Autodesk Fusion 360 part; units mm, degrees
note: some values were not read from the file. Chosen so that the rebuilt part matches the saved one: which bodies a step acts on. Set by a fixed rule: which sketch regions a step uses.
(part 2 of 3)
  line L946 (0.5127, -14.5835) -> (0.5127, -14.573)
  line L947 (0.9043, -14.7211) -> (1.0101, -14.52)
  line L948 (0.5074, -14.5941) -> (0.4915, -14.6153)
  line L949 (0.4915, -14.6153) -> (0.4809, -14.6259)
  line L950 (0.4809, -14.6259) -> (0.4598, -14.6312)
  line L951 (0.4598, -14.6312) -> (0.4439, -14.6206)
  line L952 (0.4439, -14.6206) -> (0.4227, -14.6047)
  line L953 (0.8778, -14.6047) -> (0.899, -14.5888)
  line L954 (0.899, -14.5888) -> (0.9148, -14.5677)
  line L955 (0.8778, -14.6047) -> (0.8566, -14.6259)
  line L956 (0.8566, -14.6259) -> (0.8355, -14.6312)
  line L957 (0.8355, -14.6312) -> (0.8196, -14.6259)
  line L958 (0.8196, -14.6259) -> (0.809, -14.6153)
  line L959 (0.809, -14.6153) -> (0.7931, -14.5941)
  line L960 (0.9043, -14.7211) -> (0.7296, -14.7211)
  line L961 (0.5709, -14.7211) -> (0.3963, -14.7211)
  line L962 (1.0101, -14.52) -> (0.9783, -14.52)
  line L963 (0.7138, -14.52) -> (0.5868, -14.52)
  line L964 (0.3222, -14.52) -> (0.2904, -14.52)
  line L965 (0.9783, -14.52) -> (0.9677, -14.52)
  line L966 (0.9677, -14.52) -> (0.9519, -14.5306)
  line L967 (0.9519, -14.5306) -> (0.9148, -14.5677)
  line L968 (0.5868, -14.52) -> (0.5656, -14.52)
  line L969 (0.5656, -14.52) -> (0.5444, -14.5306)
  line L970 (0.5444, -14.5306) -> (0.5127, -14.573)
  line L971 (14.0223, -13.8004) -> (14.0223, -14.0755)
  line L972 (14.0223, -14.2396) -> (14.0223, -14.52)
  line L973 (13.9905, -14.52) -> (13.9905, -14.2396)
  line L974 (13.9905, -14.0755) -> (13.9905, -13.8004)
  line L975 (13.9323, -14.5677) -> (13.9323, -14.266)
  line L976 (13.9323, -14.102) -> (13.9323, -13.8004)
  line L977 (13.8953, -14.6047) -> (13.8953, -14.2872)
  line L978 (13.8953, -14.1232) -> (13.8953, -13.8004)
  line L979 (13.8106, -14.5941) -> (13.8106, -14.2766)
  line L980 (13.8106, -14.1179) -> (13.8106, -13.8004)
  line L981 (13.8, -13.8004) -> (13.8, -14.1073)
  line L982 (13.8, -14.266) -> (13.8, -14.573)
  line L983 (13.599, -14.52) -> (13.599, -14.2396)
  line L984 (13.599, -14.0755) -> (13.599, -13.8004)
  line L985 (13.9218, -14.7211) -> (14.0223, -14.52)
  line L986 (13.5302, -14.573) -> (13.5196, -14.5941)
  line L987 (13.5302, -14.573) -> (13.5302, -14.266)
  line L988 (13.5302, -14.1073) -> (13.5302, -13.8004)
  line L989 (13.5196, -14.5941) -> (13.5196, -14.2766)
  line L990 (13.5196, -14.1179) -> (13.5196, -13.8004)
  line L991 (13.4349, -14.6047) -> (13.4349, -14.2872)
  line L992 (13.4349, -14.1232) -> (13.4349, -13.8004)
  line L993 (13.3979, -13.8004) -> (13.3979, -14.102)
  line L994 (13.3979, -14.266) -> (13.3979, -14.5677)
  line L995 (13.3397, -13.8004) -> (13.3397, -14.0755)
  line L996 (13.3397, -14.2396) -> (13.3397, -14.52)
  line L997 (13.3079, -13.8004) -> (13.3079, -14.0755)
  line L998 (13.3079, -14.2396) -> (13.3079, -14.52)
  line L999 (13.9323, -14.5677) -> (13.9482, -14.5465)
  line L1000 (13.9482, -14.5465) -> (13.9641, -14.5306)
  line L1001 (13.9641, -14.5306) -> (13.98, -14.52)
  line L1002 (13.98, -14.52) -> (13.9905, -14.52)
  line L1003 (13.9323, -14.5677) -> (13.8953, -14.6047)
  line L1004 (13.5302, -14.573) -> (13.5407, -14.5518)
  line L1005 (13.5407, -14.5518) -> (13.5566, -14.5306)
  line L1006 (13.5566, -14.5306) -> (13.5778, -14.52)
  line L1007 (13.5778, -14.52) -> (13.599, -14.52)
  line L1008 (13.8106, -14.5941) -> (13.8, -14.573)
  line L1009 (13.4085, -14.7211) -> (13.3079, -14.52)
  line L1010 (13.8106, -14.5941) -> (13.8212, -14.6153)
  line L1011 (13.8212, -14.6153) -> (13.8371, -14.6259)
  line L1012 (13.8371, -14.6259) -> (13.853, -14.6312)
  line L1013 (13.853, -14.6312) -> (13.8741, -14.6206)
  line L1014 (13.8741, -14.6206) -> (13.8953, -14.6047)
  line L1015 (13.4349, -14.6047) -> (13.3979, -14.5677)
  line L1016 (13.4349, -14.6047) -> (13.4561, -14.6259)
  line L1017 (13.4561, -14.6259) -> (13.4773, -14.6312)
  line L1018 (13.4773, -14.6312) -> (13.4931, -14.6259)
  line L1019 (13.4931, -14.6259) -> (13.509, -14.6153)
  line L1020 (13.509, -14.6153) -> (13.5196, -14.5941)
  line L1021 (13.4085, -14.7211) -> (13.5831, -14.7211)
  line L1022 (13.7471, -14.7211) -> (13.9218, -14.7211)
  line L1023 (13.3079, -14.52) -> (13.3397, -14.52)
  line L1024 (13.599, -14.52) -> (13.7313, -14.52)
  line L1025 (13.9905, -14.52) -> (14.0223, -14.52)
  line L1026 (13.3397, -14.52) -> (13.3503, -14.52)
  line L1027 (13.3503, -14.52) -> (13.3979, -14.5677)
  line L1028 (13.7313, -14.52) -> (13.7524, -14.52)
  line L1029 (13.7524, -14.52) -> (13.7683, -14.5306)
  line L1030 (13.7683, -14.5306) -> (13.7895, -14.5518)
  line L1031 (13.7895, -14.5518) -> (13.8, -14.573)
  line L1032 (0.5285, -0.3807) -> (0.5285, -0.3966)
  line L1033 (0.5285, -0.3966) -> (0.5233, -0.4019)
  line L1034 (0.5233, -0.4019) -> (0.5233, -0.4178)
  line L1035 (0.5233, -0.4178) -> (0.518, -0.4178)
  line L1036 (0.518, -0.4178) -> (0.518, -0.4283)
  line L1037 (0.518, -0.4283) -> (0.5127, -0.4336)
  line L1038 (0.4809, -0.4707) -> (0.4756, -0.4707)
  line L1039 (0.4756, -0.4707) -> (0.4703, -0.476)
  line L1040 (0.4703, -0.476) -> (0.4598, -0.476)
  line L1041 (0.4598, -0.476) -> (0.4598, -0.4813)
  line L1042 (0.4598, -0.4813) -> (0.4386, -0.4813)
  line L1043 (0.4386, -0.4813) -> (0.4333, -0.4865)
  line L1044 (0.4333, -0.4865) -> (0.4227, -0.4865)
  line L1045 (0.5285, -0.3648) -> (0.5285, -0.3807)
  line L1046 (0.5285, -0.3648) -> (0.5285, -0.349)
  line L1047 (0.5285, -0.349) -> (0.5338, -0.3437)
  line L1048 (0.5338, -0.3437) -> (0.5338, -0.3384)
  line L1049 (0.5338, -0.3384) -> (0.5391, -0.3384)
  line L1050 (0.5391, -0.3384) -> (0.5391, -0.3331)
  line L1051 (0.5391, -0.3331) -> (0.5444, -0.3278)
  line L1052 (0.5444, -0.3278) -> (0.5497, -0.3225)
  line L1053 (0.5497, -0.3225) -> (0.555, -0.3225)
  line L1054 (0.555, -0.3225) -> (0.555, -0.3172)
  line L1055 (0.555, -0.3172) -> (0.5656, -0.3172)
  line L1056 (0.7349, -0.3172) -> (0.6767, -0.3066)
  line L1057 (0.6238, -0.3066) -> (0.5656, -0.3172)
  line L1058 (0.7349, -0.3172) -> (0.7455, -0.3172)
  line L1059 (0.7455, -0.3172) -> (0.7455, -0.3225)
  line L1060 (0.7455, -0.3225) -> (0.7561, -0.3225)
  line L1061 (0.7561, -0.3225) -> (0.7561, -0.3278)
  line L1062 (0.7561, -0.3278) -> (0.7614, -0.3331)
  line L1063 (0.7614, -0.3331) -> (0.7667, -0.3331)
  line L1064 (0.7667, -0.3331) -> (0.7667, -0.3437)
  line L1065 (0.7667, -0.3437) -> (0.772, -0.349)
  line L1066 (0.772, -0.349) -> (0.772, -0.3648)
  line L1067 (0.772, -0.3807) -> (0.772, -0.3648)
  line L1068 (0.8778, -0.4865) -> (0.8672, -0.4865)
  line L1069 (0.8672, -0.4865) -> (0.8619, -0.4812)
  line L1070 (0.8619, -0.4812) -> (0.8408, -0.4812)
  line L1071 (0.8408, -0.4812) -> (0.8408, -0.476)
  line L1072 (0.8408, -0.476) -> (0.8302, -0.476)
  line L1073 (0.8302, -0.476) -> (0.8302, -0.4707)
  line L1074 (0.8302, -0.4707) -> (0.8196, -0.4707)
  line L1075 (0.7878, -0.4336) -> (0.7878, -0.4283)
  line L1076 (0.7878, -0.4283) -> (0.7825, -0.4283)
  line L1077 (0.7825, -0.4283) -> (0.7825, -0.4177)
  line L1078 (0.7825, -0.4177) -> (0.7773, -0.4177)
  line L1079 (0.7773, -0.4177) -> (0.7773, -0.4019)
  line L1080 (0.7773, -0.4019) -> (0.772, -0.3966)
  line L1081 (0.772, -0.3966) -> (0.772, -0.3807)
  line L1082 (0.8937, -0.4865) -> (0.8778, -0.4865)
  line L1083 (0.8937, -0.4865) -> (0.9254, -0.4865)
  line L1084 (0.9254, -0.4865) -> (0.9254, -0.4918)
  line L1085 (0.9254, -0.4918) -> (0.936, -0.4918)
  line L1086 (0.936, -0.4918) -> (0.9413, -0.4971)
  line L1087 (0.9413, -0.4971) -> (0.9466, -0.4971)
  line L1088 (0.9466, -0.4971) -> (0.9519, -0.5024)
  line L1089 (0.9519, -0.5024) -> (0.9572, -0.5024)
  line L1090 (0.9572, -0.5024) -> (0.9572, -0.5077)
  line L1091 (0.9572, -0.5077) -> (0.9625, -0.5077)
  line L1092 (0.9625, -0.5077) -> (0.9625, -0.513)
  line L1093 (0.9625, -0.513) -> (0.9678, -0.513)
  line L1094 (0.9678, -0.513) -> (0.9678, -0.5183)
  line L1095 (0.9678, -0.5183) -> (0.973, -0.5183)
  line L1096 (0.973, -0.5183) -> (0.973, -0.5236)
  line L1097 (0.973, -0.5236) -> (0.9783, -0.5236)
  line L1098 (0.9783, -0.5236) -> (0.9783, -0.5289)
  line L1099 (0.9783, -0.5289) -> (0.9836, -0.5342)
  line L1100 (0.9836, -0.5342) -> (0.9836, -0.5395)
  line L1101 (0.9836, -0.5395) -> (0.9889, -0.5395)
  line L1102 (0.9889, -0.5395) -> (0.9889, -0.55)
  line L1103 (0.9889, -0.55) -> (0.9942, -0.5553)
  line L1104 (0.9942, -0.7723) -> (1.0048, -0.7194)
  line L1105 (1.0048, -0.7194) -> (1.0048, -0.6876)
  line L1106 (1.0048, -0.64) -> (1.0048, -0.6083)
  line L1107 (1.0048, -0.6083) -> (0.9942, -0.5553)
  line L1108 (0.9942, -0.7723) -> (0.9889, -0.7776)
  line L1109 (0.9889, -0.7776) -> (0.9889, -0.7882)
  line L1110 (0.9889, -0.7882) -> (0.9836, -0.7882)
  line L1111 (0.9836, -0.7882) -> (0.9836, -0.7935)
  line L1112 (0.9836, -0.7935) -> (0.9783, -0.7988)
  line L1113 (0.9783, -0.7988) -> (0.9783, -0.804)
  line L1114 (0.9783, -0.804) -> (0.973, -0.804)
  line L1115 (0.973, -0.804) -> (0.973, -0.8093)
  line L1116 (0.973, -0.8093) -> (0.9677, -0.8093)
  line L1117 (0.9677, -0.8093) -> (0.9677, -0.8146)
  line L1118 (0.9677, -0.8146) -> (0.9625, -0.8146)
  line L1119 (0.9625, -0.8146) -> (0.9625, -0.8199)
  line L1120 (0.9625, -0.8199) -> (0.9572, -0.8199)
  line L1121 (0.9572, -0.8199) -> (0.9572, -0.8252)
  line L1122 (0.9572, -0.8252) -> (0.9519, -0.8252)
  line L1123 (0.9519, -0.8252) -> (0.9466, -0.8305)
  line L1124 (0.9466, -0.8305) -> (0.9413, -0.8305)
  line L1125 (0.9413, -0.8305) -> (0.936, -0.8358)
  line L1126 (0.936, -0.8358) -> (0.9254, -0.8358)
  line L1127 (0.9254, -0.8358) -> (0.9254, -0.8411)
  line L1128 (0.9254, -0.8411) -> (0.8937, -0.8411)
  line L1129 (0.8778, -0.8411) -> (0.8937, -0.8411)
  line L1130 (0.772, -0.9469) -> (0.772, -0.931)
  line L1131 (0.772, -0.931) -> (0.7773, -0.931)
  line L1132 (0.7773, -0.931) -> (0.7773, -0.9099)
  line L1133 (0.7773, -0.9099) -> (0.7825, -0.9099)
  line L1134 (0.7825, -0.9099) -> (0.7825, -0.8993)
  line L1135 (0.7825, -0.8993) -> (0.7878, -0.8993)
  line L1136 (0.7878, -0.8993) -> (0.7878, -0.894)
  line L1137 (0.8196, -0.857) -> (0.8302, -0.857)
  line L1138 (0.8302, -0.857) -> (0.8302, -0.8517)
  line L1139 (0.8302, -0.8517) -> (0.8408, -0.8517)
  line L1140 (0.8408, -0.8517) -> (0.8408, -0.8464)
  line L1141 (0.8408, -0.8464) -> (0.8619, -0.8464)
  line L1142 (0.8619, -0.8464) -> (0.8672, -0.8411)
  line L1143 (0.8672, -0.8411) -> (0.8778, -0.8411)
  line L1144 (0.772, -0.9628) -> (0.772, -0.9469)
  line L1145 (0.772, -0.9628) -> (0.772, -0.9787)
  line L1146 (0.772, -0.9787) -> (0.7667, -0.984)
  line L1147 (0.7667, -0.984) -> (0.7667, -0.9945)
  line L1148 (0.7667, -0.9945) -> (0.7614, -0.9945)
  line L1149 (0.7614, -0.9945) -> (0.7561, -0.9998)
  line L1150 (0.7561, -0.9998) -> (0.7561, -1.0051)
  line L1151 (0.7561, -1.0051) -> (0.7455, -1.0051)
  line L1152 (0.7455, -1.0051) -> (0.7455, -1.0104)
  line L1153 (0.7455, -1.0104) -> (0.7349, -1.0104)
  line L1154 (0.5656, -1.0104) -> (0.6238, -1.021)
  line L1155 (0.6767, -1.021) -> (0.7349, -1.0104)
  line L1156 (0.5656, -1.0104) -> (0.555, -1.0104)
  line L1157 (0.555, -1.0104) -> (0.555, -1.0051)
  line L1158 (0.555, -1.0051) -> (0.5444, -1.0051)
  line L1159 (0.5444, -1.0051) -> (0.5444, -0.9998)
  line L1160 (0.5444, -0.9998) -> (0.5391, -0.9945)
  line L1161 (0.5391, -0.9945) -> (0.5338, -0.9892)
  line L1162 (0.5338, -0.9892) -> (0.5338, -0.984)
  line L1163 (0.5338, -0.984) -> (0.5285, -0.9787)
  line L1164 (0.5285, -0.9787) -> (0.5285, -0.9628)
  line L1165 (0.5285, -0.9469) -> (0.5285, -0.9628)
  line L1166 (0.4227, -0.8411) -> (0.4333, -0.8411)
  line L1167 (0.4333, -0.8411) -> (0.4386, -0.8464)
  line L1168 (0.4386, -0.8464) -> (0.4598, -0.8464)
  line L1169 (0.4598, -0.8464) -> (0.4598, -0.8517)
  line L1170 (0.4598, -0.8517) -> (0.4703, -0.8517)
  line L1171 (0.4703, -0.8517) -> (0.4703, -0.857)
  line L1172 (0.4703, -0.857) -> (0.4809, -0.857)
  line L1173 (0.5127, -0.894) -> (0.518, -0.8993)
  line L1174 (0.518, -0.8993) -> (0.518, -0.9099)
  line L1175 (0.518, -0.9099) -> (0.5233, -0.9099)
  line L1176 (0.5233, -0.9099) -> (0.5233, -0.9258)
  line L1177 (0.5233, -0.9258) -> (0.5285, -0.931)
  line L1178 (0.5285, -0.931) -> (0.5285, -0.9469)
  line L1179 (0.4068, -0.8411) -> (0.4227, -0.8411)
  line L1180 (0.4068, -0.8411) -> (0.3751, -0.8411)
  line L1181 (0.3751, -0.8411) -> (0.3751, -0.8358)
  line L1182 (0.3751, -0.8358) -> (0.3645, -0.8358)
  line L1183 (0.3645, -0.8358) -> (0.3592, -0.8305)
  line L1184 (0.3592, -0.8305) -> (0.3539, -0.8305)
  line L1185 (0.3539, -0.8305) -> (0.3486, -0.8252)
  line L1186 (0.3486, -0.8252) -> (0.3433, -0.8252)
  line L1187 (0.3433, -0.8252) -> (0.3433, -0.8199)
  line L1188 (0.3433, -0.8199) -> (0.338, -0.8199)
  line L1189 (0.338, -0.8199) -> (0.338, -0.8146)
  line L1190 (0.338, -0.8146) -> (0.3327, -0.8146)
  line L1191 (0.3327, -0.8146) -> (0.3327, -0.8093)
  line L1192 (0.3327, -0.8093) -> (0.3275, -0.8093)
  line L1193 (0.3275, -0.8093) -> (0.3275, -0.804)
  line L1194 (0.3275, -0.804) -> (0.3222, -0.804)
  line L1195 (0.3222, -0.804) -> (0.3222, -0.7935)
  line L1196 (0.3222, -0.7935) -> (0.3169, -0.7935)
  line L1197 (0.3169, -0.7935) -> (0.3169, -0.7882)
  line L1198 (0.3169, -0.7882) -> (0.3116, -0.7882)
  line L1199 (0.3116, -0.7882) -> (0.3116, -0.7776)
  line L1200 (0.3116, -0.7776) -> (0.3063, -0.7723)
  line L1201 (0.3063, -0.5553) -> (0.2957, -0.6083)
  line L1202 (0.2957, -0.6083) -> (0.2957, -0.64)
  line L1203 (0.2957, -0.6876) -> (0.2957, -0.7194)
  line L1204 (0.2957, -0.7194) -> (0.3063, -0.7723)
  line L1205 (0.3063, -0.5553) -> (0.3116, -0.55)
  line L1206 (0.3116, -0.55) -> (0.3116, -0.5395)
  line L1207 (0.3116, -0.5395) -> (0.3169, -0.5395)
  line L1208 (0.3169, -0.5395) -> (0.3169, -0.5342)
  line L1209 (0.3169, -0.5342) -> (0.3222, -0.5289)
  line L1210 (0.3222, -0.5289) -> (0.3222, -0.5236)
  line L1211 (0.3222, -0.5236) -> (0.3275, -0.5236)
  line L1212 (0.3275, -0.5236) -> (0.3275, -0.5183)
  line L1213 (0.3275, -0.5183) -> (0.3327, -0.5183)
  line L1214 (0.3327, -0.5183) -> (0.3327, -0.513)
  line L1215 (0.3327, -0.513) -> (0.338, -0.513)
  line L1216 (0.338, -0.513) -> (0.338, -0.5077)
  line L1217 (0.338, -0.5077) -> (0.3433, -0.5077)
  line L1218 (0.3433, -0.5077) -> (0.3433, -0.5024)
  line L1219 (0.3433, -0.5024) -> (0.3486, -0.5024)
  line L1220 (0.3486, -0.5024) -> (0.3539, -0.4971)
  line L1221 (0.3539, -0.4971) -> (0.3592, -0.4971)
  line L1222 (0.3592, -0.4971) -> (0.3645, -0.4918)
  line L1223 (0.3645, -0.4918) -> (0.3751, -0.4918)
  line L1224 (0.3751, -0.4918) -> (0.3751, -0.4865)
  line L1225 (0.3751, -0.4865) -> (0.4068, -0.4865)
  line L1226 (0.4227, -0.4865) -> (0.4068, -0.4865)
  line L1227 (0.9043, -0.6665) -> (0.9043, -0.6135)
  line L1228 (0.9043, -0.6135) -> (0.8884, -0.5712)
  line L1229 (0.8884, -0.5712) -> (0.8884, -0.5659)
  line L1230 (0.8672, -0.5236) -> (0.8355, -0.4865)
  line L1231 (0.8355, -0.4865) -> (0.7984, -0.4548)
  line L1232 (0.7561, -0.4283) -> (0.7085, -0.4125)
  line L1233 (0.7085, -0.4125) -> (0.6608, -0.4072)
  line L1234 (0.6132, -0.4125) -> (0.5656, -0.423)
  line L1235 (0.5656, -0.423) -> (0.5233, -0.4442)
  line L1236 (0.4809, -0.4707) -> (0.4492, -0.5077)
  line L1237 (0.4492, -0.5077) -> (0.4227, -0.5448)
  line L1238 (0.4227, -0.5448) -> (0.4227, -0.55)
  line L1239 (0.4068, -0.5924) -> (0.3963, -0.64)
  line L1240 (0.3963, -0.64) -> (0.3963, -0.6876)
  line L1241 (0.4068, -0.7352) -> (0.4227, -0.7829)
  line L1242 (0.4227, -0.7829) -> (0.4492, -0.8199)
  line L1243 (0.4492, -0.8199) -> (0.4492, -0.8252)
  line L1244 (0.4862, -0.857) -> (0.5233, -0.8834)
  line L1245 (0.5233, -0.8834) -> (0.5656, -0.9046)
  line L1246 (0.6132, -0.9152) -> (0.6608, -0.9205)
  line L1247 (0.6608, -0.9205) -> (0.7085, -0.9152)
  line L1248 (0.7085, -0.9152) -> (0.7138, -0.9099)
  line L1249 (0.7561, -0.894) -> (0.7984, -0.8728)
  line L1250 (0.7984, -0.8728) -> (0.8355, -0.8411)
  line L1251 (0.8672, -0.7987) -> (0.8884, -0.7564)
  line L1252 (0.8884, -0.7564) -> (0.9043, -0.7141)
  line L1253 (0.9043, -0.7141) -> (0.9043, -0.7088)
  line L1254 (13.5408, -0.3807) -> (13.5408, -0.4072)
  line L1255 (13.5408, -0.4072) -> (13.5355, -0.4125)
  line L1256 (13.5355, -0.4125) -> (13.5355, -0.423)
  line L1257 (13.5355, -0.423) -> (13.5302, -0.423)
  line L1258 (13.5302, -0.423) -> (13.5302, -0.4336)
  line L1259 (13.5302, -0.4336) -> (13.5249, -0.4336)
  line L1260 (13.4931, -0.4707) -> (13.4878, -0.4707)
  line L1261 (13.4878, -0.4707) -> (13.4825, -0.476)
  line L1262 (13.4825, -0.476) -> (13.4773, -0.476)
  line L1263 (13.4773, -0.476) -> (13.472, -0.4813)
  line L1264 (13.472, -0.4813) -> (13.4508, -0.4813)
  line L1265 (13.4508, -0.4813) -> (13.4508, -0.4865)
  line L1266 (13.4508, -0.4865) -> (13.4402, -0.4865)
  line L1267 (13.5408, -0.3807) -> (13.5408, -0.3542)
  line L1268 (13.5408, -0.3542) -> (13.546, -0.349)
  line L1269 (13.546, -0.349) -> (13.546, -0.3384)
  line L1270 (13.546, -0.3384) -> (13.5513, -0.3384)
  line L1271 (13.5513, -0.3384) -> (13.5513, -0.3331)
  line L1272 (13.5513, -0.3331) -> (13.5566, -0.3331)
  line L1273 (13.5566, -0.3331) -> (13.5566, -0.3278)
  line L1274 (13.5566, -0.3278) -> (13.5619, -0.3278)
  line L1275 (13.5619, -0.3278) -> (13.5619, -0.3225)
  line L1276 (13.5619, -0.3225) -> (13.5672, -0.3225)
  line L1277 (13.5672, -0.3225) -> (13.5672, -0.3172)
  line L1278 (13.5672, -0.3172) -> (13.5831, -0.3172)
  line L1279 (13.7471, -0.3172) -> (13.6942, -0.3066)
  line L1280 (13.6942, -0.3066) -> (13.6889, -0.3066)
  line L1281 (13.6413, -0.3066) -> (13.636, -0.3066)
  line L1282 (13.636, -0.3066) -> (13.5831, -0.3172)
  line L1283 (13.7471, -0.3172) -> (13.7577, -0.3172)
  line L1284 (13.7577, -0.3172) -> (13.763, -0.3225)
  line L1285 (13.763, -0.3225) -> (13.7683, -0.3225)
  line L1286 (13.7683, -0.3225) -> (13.7683, -0.3278)
  line L1287 (13.7683, -0.3278) -> (13.7736, -0.3278)
  line L1288 (13.7736, -0.3278) -> (13.7736, -0.3331)
  line L1289 (13.7736, -0.3331) -> (13.7789, -0.3331)
  line L1290 (13.7789, -0.3331) -> (13.7789, -0.3384)
  line L1291 (13.7789, -0.3384) -> (13.7842, -0.3437)
  line L1292 (13.7842, -0.3437) -> (13.7842, -0.3543)
  line L1293 (13.7842, -0.3543) -> (13.7895, -0.3595)
  line L1294 (13.7895, -0.3595) -> (13.7895, -0.3807)
  line L1295 (13.89, -0.4865) -> (13.8794, -0.4865)
  line L1296 (13.8794, -0.4865) -> (13.8794, -0.4812)
  line L1297 (13.8794, -0.4812) -> (13.8583, -0.4812)
  line L1298 (13.8583, -0.4812) -> (13.853, -0.476)
  line L1299 (13.853, -0.476) -> (13.8424, -0.476)
  line L1300 (13.8424, -0.476) -> (13.8424, -0.4707)
  line L1301 (13.8424, -0.4707) -> (13.8371, -0.4707)
  line L1302 (13.8, -0.4336) -> (13.8, -0.4283)
  line L1303 (13.8, -0.4283) -> (13.7948, -0.4283)
  line L1304 (13.7948, -0.4283) -> (13.7948, -0.4125)
  line L1305 (13.7948, -0.4125) -> (13.7895, -0.4125)
  line L1306 (13.7895, -0.4125) -> (13.7895, -0.3807)
  line L1307 (13.9112, -0.4865) -> (13.89, -0.4865)
  line L1308 (13.9112, -0.4865) -> (13.9376, -0.4865)
  line L1309 (13.9376, -0.4865) -> (13.9429, -0.4918)
  line L1310 (13.9429, -0.4918) -> (13.9535, -0.4918)
  line L1311 (13.9535, -0.4918) -> (13.9535, -0.4971)
  line L1312 (13.9535, -0.4971) -> (13.9641, -0.4971)
  line L1313 (13.9641, -0.4971) -> (13.9641, -0.5024)
  line L1314 (13.9641, -0.5024) -> (13.9694, -0.5024)
  line L1315 (13.9694, -0.5024) -> (13.9694, -0.5077)
  line L1316 (13.9694, -0.5077) -> (13.9747, -0.5077)
  line L1317 (13.9747, -0.5077) -> (13.9747, -0.513)
  line L1318 (13.9747, -0.513) -> (13.98, -0.513)
  line L1319 (13.98, -0.513) -> (13.9853, -0.5183)
  line L1320 (13.9853, -0.5183) -> (13.9853, -0.5236)
  line L1321 (13.9853, -0.5236) -> (13.9905, -0.5236)
  line L1322 (13.9905, -0.5236) -> (13.9905, -0.5289)
  line L1323 (13.9905, -0.5289) -> (13.9958, -0.5289)
  line L1324 (13.9958, -0.5289) -> (13.9958, -0.5342)
  line L1325 (13.9958, -0.5342) -> (14.0011, -0.5395)
  line L1326 (14.0011, -0.5395) -> (14.0011, -0.55)
  line L1327 (14.0011, -0.55) -> (14.0064, -0.55)
  line L1328 (14.0064, -0.55) -> (14.0064, -0.5553)
  line L1329 (14.0064, -0.7723) -> (14.017, -0.7194)
  line L1330 (14.017, -0.7194) -> (14.0223, -0.6876)
  line L1331 (14.0223, -0.64) -> (14.017, -0.6083)
  line L1332 (14.017, -0.6083) -> (14.0064, -0.5553)
  line L1333 (14.0064, -0.7723) -> (14.0064, -0.7776)
  line L1334 (14.0064, -0.7776) -> (14.0011, -0.7776)
  line L1335 (14.0011, -0.7776) -> (14.0011, -0.7882)
  line L1336 (14.0011, -0.7882) -> (13.9958, -0.7935)
  line L1337 (13.9958, -0.7935) -> (13.9958, -0.7988)
  line L1338 (13.9958, -0.7988) -> (13.9905, -0.7988)
  line L1339 (13.9905, -0.7988) -> (13.9905, -0.804)
  line L1340 (13.9905, -0.804) -> (13.9853, -0.804)
  line L1341 (13.9853, -0.804) -> (13.9853, -0.8093)
  line L1342 (13.9853, -0.8093) -> (13.98, -0.8146)
  line L1343 (13.98, -0.8146) -> (13.9747, -0.8146)
  line L1344 (13.9747, -0.8146) -> (13.9747, -0.8199)
  line L1345 (13.9747, -0.8199) -> (13.9694, -0.8199)
  line L1346 (13.9694, -0.8199) -> (13.9694, -0.8252)
  line L1347 (13.9694, -0.8252) -> (13.9641, -0.8252)
  line L1348 (13.9641, -0.8252) -> (13.9641, -0.8305)
  line L1349 (13.9641, -0.8305) -> (13.9535, -0.8305)
  line L1350 (13.9535, -0.8305) -> (13.9535, -0.8358)
  line L1351 (13.9535, -0.8358) -> (13.9429, -0.8358)
  line L1352 (13.9429, -0.8358) -> (13.9376, -0.8411)
  line L1353 (13.9376, -0.8411) -> (13.9112, -0.8411)
  line L1354 (13.89, -0.8411) -> (13.9112, -0.8411)
  line L1355 (13.7895, -0.9469) -> (13.7895, -0.9152)
  line L1356 (13.7895, -0.9152) -> (13.7948, -0.9152)
  line L1357 (13.7948, -0.9152) -> (13.7948, -0.9046)
  line L1358 (13.7948, -0.9046) -> (13.8, -0.8993)
  line L1359 (13.8, -0.8993) -> (13.8, -0.894)
  line L1360 (13.8371, -0.857) -> (13.8424, -0.857)
  line L1361 (13.8424, -0.857) -> (13.8424, -0.8517)
  line L1362 (13.8424, -0.8517) -> (13.853, -0.8517)
  line L1363 (13.853, -0.8517) -> (13.8583, -0.8464)
  line L1364 (13.8583, -0.8464) -> (13.8794, -0.8464)
  line L1365 (13.8794, -0.8464) -> (13.8794, -0.8411)
  line L1366 (13.8794, -0.8411) -> (13.89, -0.8411)
  line L1367 (13.7895, -0.9469) -> (13.7895, -0.9681)
  line L1368 (13.7895, -0.9681) -> (13.7842, -0.9734)
  line L1369 (13.7842, -0.9734) -> (13.7842, -0.984)
  line L1370 (13.7842, -0.984) -> (13.7789, -0.9893)
  line L1371 (13.7789, -0.9893) -> (13.7789, -0.9945)
  line L1372 (13.7789, -0.9945) -> (13.7736, -0.9945)
  line L1373 (13.7736, -0.9945) -> (13.7736, -0.9998)
  line L1374 (13.7736, -0.9998) -> (13.7683, -0.9998)
  line L1375 (13.7683, -0.9998) -> (13.7683, -1.0051)
  line L1376 (13.7683, -1.0051) -> (13.763, -1.0051)
  line L1377 (13.763, -1.0051) -> (13.7577, -1.0104)
  line L1378 (13.7577, -1.0104) -> (13.7471, -1.0104)
  line L1379 (13.5831, -1.0104) -> (13.636, -1.021)
  line L1380 (13.636, -1.021) -> (13.6413, -1.021)
  line L1381 (13.6889, -1.021) -> (13.6942, -1.021)
  line L1382 (13.6942, -1.021) -> (13.7471, -1.0104)
  line L1383 (13.5831, -1.0104) -> (13.5672, -1.0104)
  line L1384 (13.5672, -1.0104) -> (13.5672, -1.0051)
  line L1385 (13.5672, -1.0051) -> (13.5619, -1.0051)
  line L1386 (13.5619, -1.0051) -> (13.5619, -0.9998)
  line L1387 (13.5619, -0.9998) -> (13.5566, -0.9998)
  line L1388 (13.5566, -0.9998) -> (13.5566, -0.9945)
  line L1389 (13.5566, -0.9945) -> (13.5513, -0.9945)
  line L1390 (13.5513, -0.9945) -> (13.5513, -0.9892)
  line L1391 (13.5513, -0.9892) -> (13.546, -0.9892)
  line L1392 (13.546, -0.9892) -> (13.546, -0.9787)
  line L1393 (13.546, -0.9787) -> (13.5407, -0.9734)
  line L1394 (13.5407, -0.9734) -> (13.5407, -0.9469)
  line L1395 (13.4402, -0.8411) -> (13.4508, -0.8411)
  line L1396 (13.4508, -0.8411) -> (13.4508, -0.8464)
  line L1397 (13.4508, -0.8464) -> (13.472, -0.8464)
  line L1398 (13.472, -0.8464) -> (13.4773, -0.8517)
  line L1399 (13.4773, -0.8517) -> (13.4825, -0.8517)
  line L1400 (13.4825, -0.8517) -> (13.4878, -0.857)
  line L1401 (13.4878, -0.857) -> (13.4931, -0.857)
  line L1402 (13.5249, -0.894) -> (13.5302, -0.894)
  line L1403 (13.5302, -0.894) -> (13.5302, -0.9046)
  line L1404 (13.5302, -0.9046) -> (13.5355, -0.9046)
  line L1405 (13.5355, -0.9046) -> (13.5355, -0.9152)
  line L1406 (13.5355, -0.9152) -> (13.5408, -0.9205)
  line L1407 (13.5408, -0.9205) -> (13.5407, -0.9469)
  line L1408 (13.419, -0.8411) -> (13.4402, -0.8411)
  line L1409 (13.419, -0.8411) -> (13.3873, -0.8411)
  line L1410 (13.3873, -0.8411) -> (13.3873, -0.8358)
  line L1411 (13.3873, -0.8358) -> (13.3767, -0.8358)
  line L1412 (13.3767, -0.8358) -> (13.3767, -0.8305)
  line L1413 (13.3767, -0.8305) -> (13.3661, -0.8305)
  line L1414 (13.3661, -0.8305) -> (13.3661, -0.8252)
  line L1415 (13.3661, -0.8252) -> (13.3608, -0.8252)
  line L1416 (13.3608, -0.8252) -> (13.3608, -0.8199)
  line L1417 (13.3608, -0.8199) -> (13.3555, -0.8199)
  line L1418 (13.3555, -0.8199) -> (13.3503, -0.8146)
  line L1419 (13.3503, -0.8146) -> (13.345, -0.8146)
  line L1420 (13.345, -0.8146) -> (13.345, -0.8093)
  line L1421 (13.345, -0.8093) -> (13.3397, -0.804)
  line L1422 (13.3397, -0.804) -> (13.3397, -0.7987)
  line L1423 (13.3397, -0.7987) -> (13.3344, -0.7987)
  line L1424 (13.3344, -0.7987) -> (13.3344, -0.7935)
  line L1425 (13.3344, -0.7935) -> (13.3291, -0.7935)
  line L1426 (13.3291, -0.7935) -> (13.3291, -0.7829)
  line L1427 (13.3291, -0.7829) -> (13.3238, -0.7829)
  line L1428 (13.3238, -0.7829) -> (13.3238, -0.7723)
  line L1429 (13.3238, -0.5553) -> (13.3079, -0.6083)
  line L1430 (13.3079, -0.6083) -> (13.3079, -0.64)
  line L1431 (13.3079, -0.6876) -> (13.3079, -0.7194)
  line L1432 (13.3079, -0.7194) -> (13.3238, -0.7723)
  line L1433 (13.3238, -0.5553) -> (13.3238, -0.5447)
  line L1434 (13.3238, -0.5447) -> (13.3291, -0.5447)
  line L1435 (13.3291, -0.5447) -> (13.3291, -0.5342)
  line L1436 (13.3291, -0.5342) -> (13.3344, -0.5342)
  line L1437 (13.3344, -0.5342) -> (13.3344, -0.5289)
  line L1438 (13.3344, -0.5289) -> (13.3397, -0.5289)
  line L1439 (13.3397, -0.5289) -> (13.3397, -0.5236)
  line L1440 (13.3397, -0.5236) -> (13.345, -0.5183)
  line L1441 (13.345, -0.5183) -> (13.345, -0.513)
  line L1442 (13.345, -0.513) -> (13.3503, -0.513)
  line L1443 (13.3503, -0.513) -> (13.3555, -0.5077)
  line L1444 (13.3555, -0.5077) -> (13.3608, -0.5024)
  line L1445 (13.3608, -0.5024) -> (13.3661, -0.5024)
  line L1446 (13.3661, -0.5024) -> (13.3661, -0.4971)
  line L1447 (13.3661, -0.4971) -> (13.3767, -0.4971)
  line L1448 (13.3767, -0.4971) -> (13.3767, -0.4918)
  line L1449 (13.3767, -0.4918) -> (13.3873, -0.4918)
  line L1450 (13.3873, -0.4918) -> (13.3873, -0.4865)
  line L1451 (13.3873, -0.4865) -> (13.419, -0.4865)
  line L1452 (13.4402, -0.4865) -> (13.419, -0.4865)
  line L1453 (13.9218, -0.6665) -> (13.9165, -0.6135)
  line L1454 (13.9165, -0.6135) -> (13.9006, -0.5712)
  line L1455 (13.9006, -0.5712) -> (13.9006, -0.5659)
  line L1456 (13.8794, -0.5236) -> (13.8477, -0.4865)
  line L1457 (13.8477, -0.4865) -> (13.8106, -0.4548)
  line L1458 (13.7683, -0.4283) -> (13.726, -0.4125)
  line L1459 (13.726, -0.4125) -> (13.6783, -0.4072)
  line L1460 (13.6254, -0.4125) -> (13.5831, -0.423)
  line L1461 (13.5831, -0.423) -> (13.5355, -0.4442)
  line L1462 (13.4984, -0.4707) -> (13.4614, -0.5077)
  line L1463 (13.4614, -0.5077) -> (13.4349, -0.5448)
  line L1464 (13.4349, -0.5448) -> (13.4349, -0.55)
  line L1465 (13.419, -0.5924) -> (13.4085, -0.64)
  line L1466 (13.4085, -0.64) -> (13.4085, -0.6876)
  line L1467 (13.419, -0.7352) -> (13.4349, -0.7829)
  line L1468 (13.4349, -0.7829) -> (13.4614, -0.8199)
  line L1469 (13.4614, -0.8199) -> (13.4667, -0.8252)
  line L1470 (13.4984, -0.857) -> (13.5355, -0.8834)
  line L1471 (13.5355, -0.8834) -> (13.5831, -0.9046)
  line L1472 (13.6307, -0.9152) -> (13.6783, -0.9205)
  line L1473 (13.6783, -0.9205) -> (13.726, -0.9152)
  line L1474 (13.726, -0.9152) -> (13.726, -0.9099)
  line L1475 (13.7736, -0.894) -> (13.8106, -0.8728)
  line L1476 (13.8106, -0.8728) -> (13.8477, -0.8411)
  line L1477 (13.8477, -0.8411) -> (13.853, -0.8411)
  line L1478 (13.8794, -0.7987) -> (13.9006, -0.7564)
  line L1479 (13.9006, -0.7564) -> (13.9165, -0.7141)
  line L1480 (13.9165, -0.7141) -> (13.9165, -0.7088)
  line L1481 (-0.0006, -3.3917) -> (-0.0006, -4.7993)
  line L1482 (1.3011, -3.3917) -> (1.3011, -4.7993)
  line L1483 (1.8726, -4.6352) -> (5.2275, -4.6352)
  line L1484 (-0.0006, -4.6352) -> (1.3011, -4.6352)
  line L1485 (-0.5721, -4.54) -> (-0.5721, -4.7305)
  line L1486 (-0.5721, -4.7305) -> (-0.0006, -4.6352)
  line L1487 (1.8726, -4.54) -> (1.8726, -4.7305)
  line L1488 (1.8726, -4.7305) -> (1.3011, -4.6352)
  line L1489 (13.3899, -13.7407) -> (16.9511, -13.7407) construction
  line L1490 (16.9511, -13.7407) -> (16.9511, -12.5977) construction
  line L1491 (16.9511, -12.5977) -> (13.3899, -12.5977) construction
  line L1492 (13.3899, -12.5977) -> (13.3899, -13.7407) construction
  line L1493 (13.3475, -15.995) -> (16.8323, -15.995) construction
  line L1494 (16.8323, -15.995) -> (16.8323, -14.852) construction
  line L1495 (16.8323, -14.852) -> (13.3475, -14.852) construction
  line L1496 (13.3475, -14.852) -> (13.3475, -15.995) construction
  line L1497 (-7.3876, -32.2061) -> (-7.3876, -30.1578) construction
  line L1498 (-7.3876, -30.1578) -> (-8.5306, -30.1578) construction
  line L1499 (-8.5306, -30.1578) -> (-8.5306, -32.2061) construction
  line L1500 (-8.5306, -32.2061) -> (-7.3876, -32.2061) construction
  line L1501 (13.3264, -35.1296) -> (16.901, -35.1296) construction
  line L1502 (16.901, -35.1296) -> (16.901, -33.9866) construction
  line L1503 (16.901, -33.9866) -> (13.3264, -33.9866) construction
  line L1504 (13.3264, -33.9866) -> (13.3264, -35.1296) construction
  line L1505 (-31.7292, -60.9292) -> (-31.7292, -58.7838) construction
  line L1506 (-31.7292, -58.7838) -> (-32.8722, -58.7838) construction
  line L1507 (-32.8722, -58.7838) -> (-32.8722, -60.9292) construction
  line L1508 (-32.8722, -60.9292) -> (-31.7292, -60.9292) construction
  line L1509 (53.4689, -34.1453) -> (56.3704, -34.1453) construction
  line L1510 (56.3704, -34.1453) -> (56.3704, -33.0023) construction
  line L1511 (56.3704, -33.0023) -> (53.4689, -33.0023) construction
  line L1512 (53.4689, -33.0023) -> (53.4689, -34.1453) construction
  line L1513 (5.4524, -32.9494) -> (11.3197, -32.9494) construction
  line L1514 (11.3197, -32.9494) -> (11.3197, -31.8064) construction
  line L1515 (11.3197, -31.8064) -> (5.4524, -31.8064) construction
  line L1516 (5.4524, -31.8064) -> (5.4524, -32.9494) construction
  line L1517 (53.9028, -22.7894) -> (56.0247, -22.7894) construction
  line L1518 (56.0247, -22.7894) -> (56.0247, -21.6465) construction
  line L1519 (56.0247, -21.6465) -> (53.9028, -21.6465) construction
  line L1520 (53.9028, -21.6465) -> (53.9028, -22.7894) construction
  line L1521 (20.269, -23.5091) -> (22.4467, -23.5091) construction
  line L1522 (22.4467, -23.5091) -> (22.4467, -22.3661) construction
  line L1523 (22.4467, -22.3661) -> (20.269, -22.3661) construction
  line L1524 (20.269, -22.3661) -> (20.269, -23.5091) construction
  line L1525 (22.8087, -23.5091) -> (24.7381, -23.5091) construction
  line L1526 (24.7381, -23.5091) -> (24.7381, -22.3661) construction
  line L1527 (24.7381, -22.3661) -> (22.8087, -22.3661) construction
  line L1528 (22.8087, -22.3661) -> (22.8087, -23.5091) construction
  line L1529 (-36.407, -32.259) -> (-36.407, -30.0813) construction
  line L1530 (-36.407, -30.0813) -> (-37.55, -30.0813) construction
  line L1531 (-37.55, -30.0813) -> (-37.55, -32.259) construction
  line L1532 (-37.55, -32.259) -> (-36.407, -32.259) construction
  line L1533 (-33.8565, -32.1743) -> (-33.8565, -30.6201) construction
  line L1534 (-33.8565, -30.6201) -> (-34.7772, -30.6201) construction
  line L1535 (-34.7772, -30.6201) -> (-34.7772, -32.1743) construction
  line L1536 (-34.7772, -32.1743) -> (-33.8565, -32.1743) construction
  line L1537 (-37.0103, -34.0264) -> (-37.0103, -28.0381) construction
  line L1538 (-37.0103, -28.0381) -> (-38.0157, -28.0381) construction
  line L1539 (-38.0157, -28.0381) -> (-38.0157, -34.0264) construction
  line L1540 (-38.0157, -34.0264) -> (-37.0103, -34.0264) construction
  line L1541 (15.3901, -32.1663) -> (23.4542, -32.1663) construction
  line L1542 (23.4542, -32.1663) -> (23.4542, -30.8645) construction
  line L1543 (23.4542, -30.8645) -> (15.3901, -30.8645) construction
  line L1544 (15.3901, -30.8645) -> (15.3901, -32.1663) construction
  line L1545 (5.9604, -10.9467) -> (10.8577, -10.9467) construction
  line L1546 (10.8577, -10.9467) -> (10.8577, -9.8037) construction
  line L1547 (10.8577, -9.8037) -> (5.9604, -9.8037) construction
  line L1548 (5.9604, -9.8037) -> (5.9604, -10.9467) construction
sketch "Sketch6" plane through (0, 0, 0) normal (0, 0, 1) x (1, 0, 0)
  line L0 (0.635, 0) -> (-0.635, 0)
  line L1 (-0.635, 0) -> (-0.635, 1.535)
  line L2 (-0.635, 1.535) -> (0.635, 1.535)
  line L3 (0.635, 1.535) -> (0.635, 0)
  line L4 (0.635, 0) -> (-0.635, 1.535) construction
  line L5 (-0.635, 0) -> (0.635, 1.535) construction
  point P0 (0, 0.7675)
  dimension "d4" = 1.27
  dimension "d5" = 1.535
  constraint horizontal L0
  constraint perpendicular L0 L1
  constraint parallel L0 L2
  constraint parallel L1 L3
  constraint coincident L4 P0
  constraint coincident L5 P0
  constraint midpoint L0 origin
  measures "d4" distance of L1.end L2.end
  measures "d5" distance of L0.end L1.end
extrude "Extrude2" add sketch "Sketch6" against normal blind 1.947 makes body 1
sketch "Sketch7" plane through (0, 0, 0) normal (1, 0, 0) x (0, 1, 0)
  line L0 (1.535, 0) -> (0, 0)
  line L1 (0, 0) -> (0, -1.947)
  line L2 (0, -1.947) -> (1.535, -1.947)
  line L3 (1.535, -1.947) -> (1.535, 0)
  line L4 (-0.788, -0.3545) -> (-0.7986, -0.381)
  line L5 (0.4767, -0.3122) -> (0.4502, -0.3228)
  line L6 (-0.8251, -1.0742) -> (-0.8145, -1.0477)
  line L7 (-0.4123, -0.381) -> (-0.4229, -0.3545)
  line L8 (0.0004, -0.8467) -> (0.2809, -0.5609)
  line L9 (-0.8833, -1.1165) -> (-0.8621, -1.106)
  line L10 (-0.7034, -0.3069) -> (-0.7298, -0.3122)
  line L11 (-0.9098, -0.1005) -> (-1.0632, 0)
  line L12 (-0.2853, -0.2064) -> (-1.1214, -0.2064)
  line L13 (-1.5395, 0) -> (-1.5395, -2.0479)
  line L14 (0.2809, -0.2064) -> (0.2809, -1.9473)
  line L15 (0.0004, -1.5716) -> (0.2809, -1.2859)
  line L16 (0.4185, -0.3545) -> (0.4079, -0.381)
  line L17 (-0.2853, -1.1271) -> (0.0004, -0.8467)
  line L18 (1.1222, -1.9473) -> (1.1222, -0.2064)
  line L19 (-0.2853, -0.2064) -> (-0.2853, -1.9473)
  line L20 (0.0004, -1.2065) -> (0.2809, -0.926)
  line L21 (-0.2853, -0.7673) -> (0.0004, -0.4815)
  line L22 (-0.4229, -0.3545) -> (-0.4388, -0.3387)
  line L23 (0.4079, -0.381) -> (0.4026, -0.4075)
  line L24 (0.5031, -0.3069) -> (0.4767, -0.3122)
  line L25 (-0.7034, -0.3069) -> (-0.5076, -0.3069)
  line L26 (-0.8145, -1.0477) -> (-0.8092, -1.0213)
  line L27 (-0.4811, -0.3122) -> (-0.5076, -0.3069)
  line L28 (-0.407, -0.4075) -> (-0.4123, -0.381)
  line L29 (-0.8039, -1.0213) -> (-0.8039, -0.4075)
  line L30 (-0.841, -1.0901) -> (-0.8251, -1.0742)
  line L31 (-1.5395, -0.9313) -> (-1.1214, -0.5186)
  line L32 (0.4026, -0.4075) -> (0.4026, -1.3335)
  line L33 (-1.1214, -0.2064) -> (-1.1214, -1.9473)
  line L34 (0.4026, -1.3335) -> (0.2491, -1.5346)
  line L35 (-0.46, -0.3228) -> (-0.4811, -0.3122)
  line L36 (-0.407, -1.3335) -> (-0.2483, -1.5346)
  line L37 (-0.8621, -1.106) -> (-0.841, -1.0901)
  line L38 (-0.4388, -0.3387) -> (-0.46, -0.3228)
  line L39 (1.535, 0) -> (1.535, -2.0479)
  line L40 (-0.7986, -0.381) -> (-0.8039, -0.4075)
  line L41 (-0.7563, -0.3228) -> (-0.788, -0.3545)
  line L42 (0.4502, -0.3228) -> (0.4185, -0.3545)
  line L43 (-1.5395, -1.2965) -> (-1.1214, -0.8784)
  line L44 (-0.407, -0.4075) -> (-0.407, -1.3335)
  line L45 (-0.7298, -0.3122) -> (-0.7563, -0.3228)
  line L46 (-1.1214, -1.1271) -> (-0.9098, -1.1271)
  line L47 (-0.9098, -1.1218) -> (-0.8833, -1.1165)
  line L48 (0.8524, -1.106) -> (0.8788, -1.1165)
  line L49 (-1.5395, 0) -> (1.535, 0)
  line L50 (-0.4758, -1.8415) -> (-0.968, -1.8415)
  line L51 (0.3655, -1.5769) -> (0.355, -1.5557)
  line L52 (0.0004, -1.8468) -> (0.0004, -3.2173)
  line L53 (0.2809, -0.2064) -> (1.1222, -0.2064)
  line L54 (-1.1214, -1.9473) -> (1.1222, -1.9473)
  line L55 (-1.5395, -2.0214) -> (-1.1214, -1.6034)
  line L56 (-1.2061, -2.2013) -> (-1.1585, -2.196)
  line L57 (0.9053, -0.1005) -> (0.9053, -0.2064)
  line L58 (-1.2061, -2.0479) -> (-1.1849, -2.0426)
  line L59 (1.2016, -2.2013) -> (2.5616, -2.2013)
  line L60 (-1.2061, -2.2013) -> (-2.566, -2.2013)
  line L61 (-1.1585, -2.196) -> (-1.1161, -2.1855)
  line L62 (-0.0843, -2.9686) -> (-0.2589, -2.9686)
  line L63 (-2.566, -2.2013) -> (-2.566, -2.0479)
  line L64 (-1.042, -2.1325) -> (-1.0103, -2.0955)
  line L65 (-1.2378, -2.0479) -> (-1.1214, -1.9473)
  line L66 (-2.566, -2.0479) -> (-1.2061, -2.0479)
  line L67 (-0.1478, -2.7675) -> (-0.1689, -2.7675)
  line L68 (1.1222, -1.8944) -> (1.535, -1.4817)
  line L69 (-1.1373, -2.0055) -> (-1.132, -1.9897)
  line L70 (-0.9891, -2.0585) -> (-0.9785, -2.0161)
  line L71 (0.2015, -2.2966) -> (0.2015, -1.9473)
  line L72 (-0.968, -1.8415) -> (-0.968, -1.9685)
  line L73 (-1.169, -2.0373) -> (-1.1479, -2.0267)
  line L74 (1.0058, -2.0955) -> (1.0376, -2.1325)
  line L75 (-0.3594, -2.4395) -> (-0.3594, -2.7675)
  line L76 (-1.5395, -2.0479) -> (-1.2378, -2.0479)
  line L77 (1.1117, -2.1855) -> (1.154, -2.196)
  line L78 (-0.3912, -1.7886) -> (-0.3806, -1.7674)
  line L79 (0.4767, -1.8415) -> (0.9688, -1.8415)
  line L80 (-0.2165, -2.8522) -> (-0.2165, -2.4818)
  line L81 (-1.1849, -2.0426) -> (-1.169, -2.0373)
  line L82 (-1.0103, -2.0955) -> (-0.9891, -2.0585)
  line L83 (-1.0791, -2.1643) -> (-1.042, -2.1325)
  line L84 (0.3708, -1.5981) -> (0.3708, -1.741)
  line L85 (-0.3753, -1.5981) -> (-0.3753, -1.741)
  line L86 (1.2334, -2.0479) -> (1.1222, -1.9473)
  line L87 (-1.1479, -2.0267) -> (-1.1373, -2.0055)
  line L88 (-1.1161, -2.1855) -> (-1.0791, -2.1643)
  line L89 (-0.3541, -1.5558) -> (-0.3647, -1.5769)
  line L90 (-1.132, -1.9897) -> (-1.1267, -1.9685)
  line L91 (0.2491, -1.5346) -> (0.3126, -1.5346)
  line L92 (2.5616, -2.2013) -> (2.5616, -2.0479)
  line L93 (0.4079, -1.8098) -> (0.4237, -1.8256)
  line L94 (-0.9785, -2.0161) -> (-0.9733, -1.9685)
  line L95 (0.1803, -2.7781) -> (0.175, -2.7728)
  line L96 (1.535, -2.0479) -> (1.2334, -2.0479)
  line L97 (0.3814, -1.7674) -> (0.392, -1.7886)
  line L98 (0.1856, -2.7834) -> (0.1803, -2.7781)
  line L99 (-0.3806, -1.7674) -> (-0.3753, -1.741)
  line L100 (-0.2853, -2.3125) -> (-0.2853, -1.9473)
  line L101 (1.0376, -2.1325) -> (1.0746, -2.1643)
  line L102 (1.1593, -2.0373) -> (1.2016, -2.0479)
  line L103 (0.9847, -2.0585) -> (1.0058, -2.0955)
  line L104 (0.302, -1.9473) -> (0.302, -2.3019)
  line L105 (-0.3541, -2.2754) -> (-0.3541, -1.9473)
  line L106 (-0.2853, -0.4022) -> (0.0004, -0.1217)
  line L107 (-0.9098, -0.2064) -> (-0.9098, -0.1005)
  line L108 (0.0004, 0.291) -> (0.0004, -1.0795)
  line L109 (0.0004, -0.4815) -> (0.3867, -0.0953)
  line L110 (-1.5395, -0.5715) -> (-1.005, -0.037)
  line L111 (0.0004, -1.3335) -> (0.0004, -1.5928)
  line L112 (-0.2853, -1.487) -> (0.0004, -1.2065)
  line L113 (0.392, -0.1005) -> (0.2385, 0)
  line L114 (-0.3965, -0.1535) -> (-0.243, 0)
  line L115 (-0.3965, -0.1005) -> (-0.9098, -0.1005)
  line L116 (-0.243, 0) -> (-0.3965, -0.1005)
  line L117 (0.0004, -0.1217) -> (0.1221, 0)
  line L118 (-1.5395, -0.2064) -> (-1.3278, 0)
  line L119 (0.392, -0.2064) -> (0.392, -0.1005)
  line L120 (-0.3965, -0.1005) -> (-0.3965, -0.2064)
  line L121 (0.8365, -1.0901) -> (0.8524, -1.106)
  line L122 (1.1222, -1.9685) -> (1.1222, -1.1271)
  line L123 (0.9053, -0.1005) -> (1.0587, 0)
  line L124 (0.81, -1.0477) -> (0.8206, -1.0689)
  line L125 (-1.5395, -1.6563) -> (-1.1214, -1.2435)
  line L126 (1.1222, -1.5346) -> (1.535, -1.1218)
  line L127 (0.392, -0.1005) -> (0.9053, -0.1005)
  line L128 (-1.1214, -1.9685) -> (-1.1214, -1.1271)
  line L129 (0.6989, -0.3069) -> (0.5031, -0.3069)
  line L130 (0.355, -1.9473) -> (0.355, -2.2754)
  line L131 (0.2544, -2.9686) -> (0.0798, -2.9686)
  line L132 (0.355, -1.5557) -> (0.3338, -1.5452)
  line L133 (0.3708, -1.5981) -> (0.3655, -1.5769)
  line L134 (0.3497, -1.9473) -> (0.3497, -2.2754)
  line L135 (-0.3488, -2.7675) -> (-0.3541, -2.7675)
  line L136 (-0.1689, -2.7675) -> (-0.1742, -2.7728)
  line L137 (0.355, -2.7675) -> (0.2544, -2.9686)
  line L138 (0.4237, -1.8256) -> (0.4502, -1.8362)
  line L139 (-0.2853, -2.8416) -> (-0.2853, -2.4765)
  line L140 (-0.206, -2.4606) -> (-0.206, -2.8152)
  line L141 (0.4502, -1.8362) -> (0.4767, -1.8415)
  line L142 (-0.0155, -1.9473) -> (0.0004, -1.9315)
  line L143 (0.1698, -2.7675) -> (0.1486, -2.7675)
  line L144 (-0.3647, -1.5769) -> (-0.37, -1.5981)
  line L145 (-0.3118, -1.5399) -> (-0.333, -1.5452)
  line L146 (0.7677, -0.3387) -> (0.7465, -0.3228)
  line L147 (1.3286, -2.0479) -> (1.535, -1.8415)
  line L148 (0.7836, -0.3545) -> (0.7677, -0.3387)
  line L149 (0.1486, -2.7675) -> (-0.1478, -2.7675)
  line L150 (-0.2483, -1.5346) -> (-0.3118, -1.5346)
  line L151 (0.8047, -1.0213) -> (0.8047, -0.4075)
  line L152 (0.9688, -1.8415) -> (0.9688, -1.9685)
  line L153 (0.0004, -1.9315) -> (0.2809, -1.651)
  line L154 (-0.206, -1.9473) -> (-0.206, -2.2966)
  line L155 (-0.4758, -1.8415) -> (-0.4494, -1.8362)
  line L156 (0.2862, -2.3125) -> (0.2862, -1.9473)
  line L157 (-0.2165, -2.3177) -> (-0.2165, -1.9473)
  line L158 (0.355, -2.7675) -> (0.3497, -2.7675)
  line L159 (-0.1477, -2.4395) -> (-0.1478, -2.7675)
  line L160 (-0.3541, -2.7675) -> (-0.3541, -2.4395)
  line L161 (0.3761, -1.741) -> (0.3814, -1.7674)
  line L162 (-0.3594, -1.9473) -> (-0.3594, -2.2754)
  line L163 (0.355, -2.4395) -> (0.355, -2.7675)
  line L164 (0.2227, -2.8681) -> (0.2174, -2.8681)
  line L165 (-0.1477, -1.9473) -> (-0.1477, -2.2754)
  line L166 (0.9741, -2.0161) -> (0.9847, -2.0585)
  line L167 (-0.4494, -1.8362) -> (-0.4229, -1.8256)
  line L168 (0.3338, -1.5452) -> (0.3126, -1.5399)
  line L169 (1.1328, -2.0055) -> (1.1434, -2.0267)
  line L170 (0.7942, -0.381) -> (0.7836, -0.3545)
  line L171 (0.1486, -2.7675) -> (0.1486, -2.4395)
  line L172 (-0.2853, -1.8521) -> (0.0004, -1.5716)
  line L173 (0.1698, -2.7728) -> (0.1698, -2.7675)
  line L174 (1.1222, -1.1271) -> (0.9053, -1.1271)
  line L175 (-0.3012, -2.3019) -> (-0.3012, -1.9473)
  line L176 (0.2015, -2.8152) -> (0.2015, -2.4606)
  line L177 (-0.3488, -2.7728) -> (-0.3488, -2.7675)
  line L178 (0.2121, -2.8522) -> (0.2121, -2.4818)
  line L179 (-0.3541, -2.7675) -> (-0.3594, -2.7675)
  line L180 (0.302, -2.4659) -> (0.302, -2.8205)
  line L181 (-0.333, -1.5452) -> (-0.3541, -1.5558)
  line L182 (0.7465, -0.3228) -> (0.7254, -0.3122)
  line L183 (0.1486, -2.2754) -> (0.1486, -1.9473)
  line L184 (-0.4229, -1.8256) -> (-0.407, -1.8097)
  line L185 (0.175, -2.7728) -> (0.1698, -2.7728)
  line L186 (-0.2589, -2.9686) -> (-0.3594, -2.7675)
  line L187 (0.2121, -2.3177) -> (0.2121, -1.9473)
  line L188 (-0.407, -1.8097) -> (-0.3912, -1.7886)
  line L189 (0.3497, -2.7675) -> (0.3444, -2.7675)
  line L190 (-0.3171, -2.8046) -> (-0.3171, -2.7993)
  line L191 (1.1275, -1.9897) -> (1.1328, -2.0055)
  line L192 (1.0005, -0.2064) -> (1.2069, 0)
  line L193 (0.2491, -2.8734) -> (0.2438, -2.8787)
  line L194 (0.9688, -1.9685) -> (0.9741, -2.0161)
  line L195 (-0.2218, -2.8681) -> (-0.2271, -2.8681)
  line L196 (0.2809, -2.8469) -> (0.2756, -2.8522)
  line L197 (-0.3224, -2.7993) -> (-0.3224, -2.794)
  line L198 (-0.2324, -2.8787) -> (-0.2483, -2.8787)
  line L199 (0.8206, -1.0689) -> (0.8365, -1.0901)
  line L200 (1.1434, -2.0267) -> (1.1593, -2.0373)
  line L201 (0.2703, -2.8575) -> (0.2597, -2.8681)
  line L202 (0.228, -2.8787) -> (0.228, -2.8734)
  line L203 (-0.3012, -2.8205) -> (-0.3012, -2.4659)
  line L204 (0.8788, -1.1165) -> (0.9053, -1.1218)
  line L205 (1.1222, -0.8096) -> (1.535, -0.3969)
  line L206 (-0.28, -2.8469) -> (-0.2853, -2.8469)
  line L207 (0.2174, -2.8575) -> (0.2121, -2.8522)
  line L208 (1.0746, -2.1643) -> (1.1117, -2.1855)
  line L209 (1.154, -2.196) -> (1.2016, -2.2013)
  line L210 (0.3444, -2.7675) -> (0.3444, -2.7728)
  line L211 (0.2174, -2.8681) -> (0.2174, -2.8575)
  line L212 (2.5616, -2.0479) -> (1.2016, -2.0479)
  line L213 (0.3497, -2.4395) -> (0.3497, -2.7675)
  line L214 (0.2544, -2.8681) -> (0.2544, -2.8734)
  line L215 (0.2862, -2.8416) -> (0.2862, -2.4765)
  line L216 (0.2121, -2.8522) -> (0.2015, -2.8152)
  line L217 (1.1222, -1.1748) -> (1.535, -0.7567)
  line L218 (-0.3224, -2.794) -> (-0.333, -2.7834)
  line L219 (0.2015, -2.8152) -> (0.2015, -2.8099)
  line L220 (-0.2218, -2.8575) -> (-0.2218, -2.8681)
  line L221 (0.2597, -2.8681) -> (0.2544, -2.8681)
  line L222 (0.2544, -2.8734) -> (0.2491, -2.8734)
  line L223 (1.1222, -0.4498) -> (1.535, -0.0318)
  line L224 (0.1909, -2.7887) -> (0.1856, -2.7887)
  line L225 (0.3179, -2.794) -> (0.3179, -2.7993)
  line L226 (-0.3382, -2.7781) -> (-0.3435, -2.7728)
  line L227 (0.1962, -2.7993) -> (0.1909, -2.794)
  line L228 (-0.2483, -2.8787) -> (-0.2483, -2.8734)
  line L229 (-0.2165, -2.8575) -> (-0.2218, -2.8575)
  line L230 (0.2015, -2.8099) -> (0.1962, -2.8046)
  line L231 (-0.1795, -2.7728) -> (-0.1795, -2.7781)
  line L232 (-0.1901, -2.7834) -> (-0.1901, -2.7887)
  line L233 (0.2756, -2.8522) -> (0.2703, -2.8575)
  line L234 (0.3285, -2.7834) -> (0.3285, -2.7887)
  line L235 (0.3391, -2.7728) -> (0.3338, -2.7781)
  line L236 (-0.3065, -2.8152) -> (-0.3118, -2.8152)
  line L237 (0.3232, -2.7887) -> (0.3179, -2.794)
  line L238 (-0.2853, -2.8469) -> (-0.2853, -2.8416)
  line L239 (0.2438, -2.8787) -> (0.228, -2.8787)
  line L240 (0.1856, -2.7887) -> (0.1856, -2.7834)
  line L241 (-0.3012, -2.8205) -> (-0.2853, -2.8416)
  line L242 (0.392, -1.7886) -> (0.4079, -1.8098)
  line L243 (-0.2165, -2.8522) -> (-0.2165, -2.8575)
  line L244 (-0.1848, -2.7834) -> (-0.1901, -2.7834)
  line L245 (-0.1795, -2.7781) -> (-0.1848, -2.7781)
  line L246 (-0.1954, -2.794) -> (-0.2007, -2.7993)
  line L247 (0.3126, -2.8046) -> (0.3073, -2.8099)
  line L248 (-0.2007, -2.7993) -> (-0.2007, -2.8099)
  line L249 (-0.2589, -2.8734) -> (-0.2589, -2.8681)
  line L250 (-0.2271, -2.8734) -> (-0.2324, -2.8734)
  line L251 (-0.206, -2.8099) -> (-0.206, -2.8152)
  line L252 (-0.1954, -2.7887) -> (-0.1954, -2.794)
  line L253 (0.1962, -2.8046) -> (0.1962, -2.7993)
  line L254 (0.3285, -2.7887) -> (0.3232, -2.7887)
  line L255 (0.228, -2.8734) -> (0.2227, -2.8734)
  line L256 (0.3126, -2.7993) -> (0.3126, -2.8046)
  line L257 (-0.1742, -2.7728) -> (-0.1795, -2.7728)
  line L258 (-0.3012, -2.8205) -> (-0.3065, -2.8152)
  line L259 (0.1909, -2.794) -> (0.1909, -2.7887)
  line L260 (0.2227, -2.8734) -> (0.2227, -2.8681)
  line L261 (0.7995, -0.4075) -> (0.7942, -0.381)
  line L262 (-0.1848, -2.7781) -> (-0.1848, -2.7834)
  line L263 (0.3073, -2.8099) -> (0.3073, -2.8152)
  line L264 (-0.2747, -2.8575) -> (-0.28, -2.8522)
  line L265 (-0.2483, -2.8734) -> (-0.2589, -2.8734)
  line L266 (1.1222, -1.9685) -> (1.1275, -1.9897)
  line L267 (0.2862, -2.8416) -> (0.302, -2.8205)
  line L268 (-0.2589, -2.8681) -> (-0.2642, -2.8681)
  line L269 (-0.2324, -2.8734) -> (-0.2324, -2.8787)
  line L270 (-0.2271, -2.8681) -> (-0.2271, -2.8734)
  line L271 (-0.3118, -2.8099) -> (-0.3171, -2.8046)
  line L272 (0.3338, -2.7781) -> (0.3285, -2.7834)
  line L273 (0.302, -2.8152) -> (0.302, -2.8205)
  line L274 (0.8047, -1.0213) -> (0.81, -1.0477)
  line L275 (-0.2642, -2.8681) -> (-0.2747, -2.8575)
  line L276 (-0.3171, -2.7993) -> (-0.3224, -2.7993)
  line L277 (-0.3435, -2.7728) -> (-0.3488, -2.7728)
  line L278 (-0.333, -2.7834) -> (-0.3382, -2.7781)
  line L279 (-0.28, -2.8522) -> (-0.28, -2.8469)
  line L280 (0.3073, -2.8152) -> (0.302, -2.8152)
  line L281 (-0.1901, -2.7887) -> (-0.1954, -2.7887)
  line L282 (-0.2165, -2.8522) -> (-0.206, -2.8152)
  line L283 (0.2862, -2.8416) -> (0.2809, -2.8416)
  line L284 (0.7254, -0.3122) -> (0.6989, -0.3069)
  line L285 (-0.2007, -2.8099) -> (-0.206, -2.8099)
  line L286 (0.3179, -2.7993) -> (0.3126, -2.7993)
  line L287 (0.3444, -2.7728) -> (0.3391, -2.7728)
  line L288 (-0.3118, -2.8152) -> (-0.3118, -2.8099)
  line L289 (0.2809, -2.8416) -> (0.2809, -2.8469)
  line L290 (0.6486, -0.1005) -> (0.6486, 0.15)
  line L291 (0.3126, -1.5346) -> (0.3338, -1.5452)
  line L292 (0.3761, -1.741) -> (0.3708, -1.7089)
  line L293 (0.8788, -1.1165) -> (0.9053, -1.1271)
  line L294 (0.7995, -0.4075) -> (0.8047, -0.4563)
  constraint midpoint L127 L290.start
  constraint perpendicular L0 L290
  constraint coincident L91.end L291.start
  constraint coincident L132.end L168.start
  constraint parallel L132 L291
  constraint coincident L161.start L292.start
  constraint coincident L84 L292.end
  constraint coincident L48.end L204.start
  constraint coincident L174.end L293.end
  constraint coincident L261.start L294.start
  constraint coincident L151 L294.end
ref_plane "WorkPlane1" through (0, 0.6486, 0.0247) normal (0, 1, 0) x (0, 0, 1)